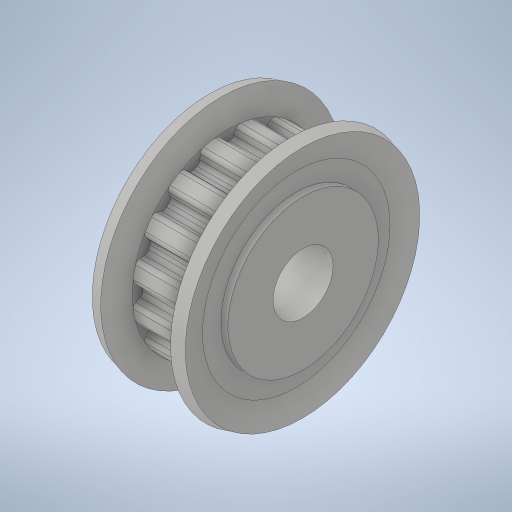
# Autodesk Inventor part: 3d_ATP16XL025-A-H8_b
Saved by Autodesk Inventor 2023 (Build 270158000, 158)
## iProperties
Category: PARTsolutions
Company: MISUMI
Created: 2023-01-14
Part Number: 3d_ATP16XL025-A-H8_b
Material: Generic
Catalog Web Link: www.cadenas.de
Description: ATP__XL025, ATP__XL031, ATP__ XL037, ATP__XL050, BTP__XL025, BTP__XL031, BTP__XL037, BTP__XL050, KTP__XL025, KTP__XL031, KTP__ XL037, KTP__XL050, NTP__XL025, NTP__XL031, NTP__ XL037, NTP__XL050, MTP__XL025, MTP__ XL037, MTP__XL050, MTPB__XL025, MTPB__ XL037, MTPB__XL050, MTPP__XL025, MTPP__ XL037, MTPP__XL050, STP__XL025, STP__ XL037, STP__XL050, KATP__XL025, KATP__XL031, KATP__ XL037, KATP__XL050, KKTP__XL025, KKTP__XL031, KKTP__ XL037, KKTP__XL050_body-Timing Pulleys XL Type
Vendor: MISUMI
Document SubType Name: Modeling
Designer: psAdmin
Manufacturer: MISUMI
Mass: 5.94338 g
Surface Area: 36.4815 cm^2
Volume: 5.94338 cm^3
Density: 1 g/cm^3
Appearance: PSOLRGB-175-175-175
PSOL_IDENT_0: {$CADENAS_DATA/23d-libs/misumi/metric/51_timing_pulleys/mtp_xl/mtp_xl.prj},873 {VTYP=3D},{NB=ATP16XL
PSOL_IDENT_1: 025-A-H8_b},{LINA=ATP16XL025-A-H8},{NN=ATP__XL025, ATP__XL031, ATP__ XL037, ATP__XL050, BTP__XL025,
PSOL_IDENT_2: BTP__XL031, BTP__XL037, BTP__XL050, KTP__XL025, KTP__XL031, KTP__ XL037, KTP__XL050, NTP__XL025, NTP
PSOL_IDENT_3: __XL031, NTP__ XL037, NTP__XL050, MTP__XL025, MTP__ XL037, MTP__XL050, MTPB__XL025, MTPB__ XL037, MT
PSOL_IDENT_4: PB__XL050, MTPP__XL025, MTPP__ XL037, MTPP__XL050, STP__XL025, STP__ XL037, STP__XL050, KATP__XL025,
PSOL_IDENT_5: KATP__XL031, KATP__ XL037, KATP__XL050, KKTP__XL025, KKTP__XL031, KKTP__ XL037, KKTP__XL050_body},{
PSOL_IDENT_6: DATE=25.04.2022 01:23:04},{GEOMDATE=17.11.2021 02:38:37},{VERSION=},{LINEID=30},{WBVAR=MATP,ST,TNW,P
PSOL_IDENT_7: S,SBS,DD,Z,J,Q,R,S,T,ALT1,ALT2,M,QSC,QFC,QTC,ALT3,K,KSC,KFC,KTC,ALT4,ZM,ZSC,ZFC,ZTC,ALT5,ALT6,ALT7,F
PSOL_IDENT_8: C,ALT8,SRG,ALT9,BTC,TL,ALT10,TPC,ALT11,BC,ALT12,SLH,ALT13,BN},{WBNUMERIC=DD,Z,J,Q,R,S,T,QSC,QFC,QTC,
PSOL_IDENT_9: K,KSC,KFC,KTC,ZSC,ZFC,ZTC,FC,SRG,BTC,TL,BC,SLH,BN}  {NB=ATP16XL025-A-H8_b},{LINA=ATP16XL025-A-H8},{K
PSOL_IDENT_10: T=DUMMY},{PN=ATP16XL025-A-H8},{TYPE=ATP},{MATP=A2017},{MATPALG= 'A2017','Aluminum Alloy 2000 series'
PSOL_IDENT_11: ,'S45C','1045 Carbon Steel Equivalent','SUS304','SUS304', 'A6000', '6000 Series Aluminum Alloy' },{S
PSOL_IDENT_12: T=CA},{STALG= 'CA','Clear Anodize','BA','Black Anodize','HAT','Hard Clear Anodize','ENP','Electroles
PSOL_IDENT_13: s Nickel Plating' },{NT=16},{TNW=XL025},{TNWALG= 'XL025','XL031','XL037','XL050' },{BW=6.4mm (1/4inc
PSOL_IDENT_14: h)},{PS=A},{PSALG= 'A','B' },{SBS=H},{SBSALG= 'H','Round Hole','P','Round Hole + Tap','N','New JIS K
PSOL_IDENT_15: eywayed Bore + Tap (Standard)','NK','New JIS Keywayed Bore + Tap (width 4.0mm, height 1.8mm)','C','O
PSOL_IDENT_16: ld JIS Keywayed Bore + Tap','V','Stepped Hole','Y','Both Ends Stepped Hole','WB','Double Stepped Hol
PSOL_IDENT_17: e' },{DD=8.00},{DDALG=[5:6/1],6.35,[7:12/1],12.7,[13:16/1]},{DDHA=[5:6/1],6.35,[7:12/1],12.7,[13:16/
PSOL_IDENT_18: 1]},{DDPA=[5:6/1],6.35,[7:12/1],12.7,[13:13/1]},{DDNA=[8:8/1],[10:13/1]},{DDNK=[10:10/1]},{DDCA=[10,
PSOL_IDENT_19: 12]},{DDVA=[5:6/1],6.35,[7:12/1],12.7,[13:14/1]},{DDY=[5:14/1]},{DDWB=[5:12/1]},{DDHB=},{DDPB=},{DDN
PSOL_IDENT_20: B=},{DDCB=},{DDVFB=},{Z=0},{ZALG=[0]},{ZMIN=10.000},{ZAMAX=16.000},{ZBMAX=0.000},{DDZ=8.000},{J=0.0}
PSOL_IDENT_21: ,{JALG=[0]},{JMIN=2.000},{JMAX=10.5},{JPN=},{Q=0},{QALG=[0]},{QRMIN=10.000},{QRMAX=16},{WBQMIN=12.00
PSOL_IDENT_22: 0},{R=0},{RALG=[0]},{WBRMAX=-2.000},{S=0.0},{SALG=[0]},{SMAX=6.5},{T=0.0},{TALG=[0]},{TMAX=8},{SBSPN=
PSOL_IDENT_23: -H8},{A=7.5},{W=12.5},{L=0},{PD=25.87},{OD=25.36},{D=0},{DALG=17.000},{DE=20},{F=32},{E=20},{TT=1.6}
PSOL_IDENT_24: ,{BBK=0.000},{TTK=0.0},{ALT1=},{ANG=112.500},{ALT1ALG= '','Not applicable' },{ALT1PN=},{ALT2=},{ALT2
PSOL_IDENT_25: ALG= '','Not applicable' },{M=N/A},{MALG= 'N/A' },{MFTALG= 'N/A' },{MSALG= 'N/A' },{M3D=0.000},{KDML=
PSOL_IDENT_26: 0.000},{ML=0.000},{MUL=0.000},{PITCH=0.000},{QSC=0.0},{QSCALG=0},{QFC=0.0},{QFCALG=0},{QTC=0.0},{QTC
PSOL_IDENT_27: ALG=0},{QPCDMIN=0.000},{QPCDMINALG=0.000},{QPCDMAX=16.000},{ALT2PN=},{TAP=0.000},{ALT3=},{ALT3ALG= ''
PSOL_IDENT_28: ,'Not applicable' },{K=0.0},{KALG=0},{KMIN=4.000},{KFTMAX=0.000},{KSMAX=0.000},{KSC=0.0},{KSCALG=0},
PSOL_IDENT_29: {KFC=0.0},{KFCALG=0},{KTC=0.0},{KTCALG=0},{KSCMIN=12.000},{KPCDMIN=12.000},{KPCDMAX=16.000},{ALT3PN=
PSOL_IDENT_30: },{ALT4=},{ALT4ALG= '','Not applicable' },{ALT4MIN=18.500},{ALT4MAX=9.500},{ZM=N/A},{ZMALG= 'N/A' },
PSOL_IDENT_31: {ZMFTALG= 'N/A' },{ZMSALG= 'N/A' },{ZMDD1=0.0},{ZMDD2=0.0},{ZMHH=0.0},{ZSC=0.0},{ZSCALG=[0]},{ZFC=0.
PSOL_IDENT_32: 0},{ZFCALG=[0]},{ZTC=0.0},{ZTCALG=[0]},{ZPCDMIN=0.000},{ZPCDMINALG=0.000},{ZPCDMAX=16.000},{ALT4PN=}
PSOL_IDENT_33: ,{ALT5=},{ALT5ALG= '','w/o Flange not Attached','NFC','with NFC (Flange not Attached)' },{ALT5PN=},{
PSOL_IDENT_34: ALT6=},{ALT6ALG= '','w/o Flange Attached on One Side Only','RFC','with RFC (Flange Attached on The B
PSOL_IDENT_35: oss Side Only)','LFC','with LFC (Flange Attached on The Opposite Side Only)' },{ALT6PN=},{ALT7=},{AL
PSOL_IDENT_36: T7ALG= '','w/o FC (Flange Cut)','FC','with FC (Flange Cut)' },{FC=0.0},{FCALG=0},{FCMIN=26.5},{FCMAX=
PSOL_IDENT_37: 30.0},{ALT7PN=},{ALT8=},{ALT8ALG= '','Not applicable' },{ALT8ALGALG=16.000},{ALT8DD2=0.000},{ALT8MM=
PSOL_IDENT_38: 0.000},{ALT8NN=0.000},{QC=0.000},{KC=0.000},{ZC=0.000},{SRG=0.0},{SRGALG=[0]},{SRGMAX=0.000},{DD2=0.
PSOL_IDENT_39: 0},{MM=0.00},{NN=0.00},{ALT8PN=},{ALT9=},{ALT9ALG= '','w/o BTC (Taper for Bearing Holder)','BTC','wi
PSOL_IDENT_40: th BTC (Taper for Bearing Holder)' },{BTC9=9.000},{TL9=1.000},{BTC=0},{BTCALG=[0]},{TL=0.0},{TLALG=0
PSOL_IDENT_41: },{TLMIN=1.000},{TLMAX=-13.000},{BTCL=0},{BTCD=0},{ALT9PN=},{WLBCTL=12.500},{ALT10=},{ALT10ALG= '','
PSOL_IDENT_42: Not applicable' },{TPC=N/A},{TPCALG= 'N/A' },{TPCM=4.000},{ALT10PN=},{ALT11=},{ALT11ALG= '','Not app
PSOL_IDENT_43: licable' },{BC=0.0},{BCALG=0},{BCMIN=3},{BCMAX=-13},{M1WBC=6.25},{ALT11PN=},{KTT=8.68},{ALT12=},{ALT
PSOL_IDENT_44: 12ALG= '','Not applicable' },{SLHALG=[0]},{SLH=0},{ALT12PN=},{ALT13=},{ALT13ALG= '', 'Not applicable'
PSOL_IDENT_45: },{BN=0.0},{BNALG=0},{BNMIN=-12},{BNMAX=-2.5},{ALT13PN=},{AC=-},{M1=4.000},{M1L=3.000},{KEYA=0.000}
PSOL_IDENT_46: ,{KEYB=0.000},{KEYM=0.000}
NB: ATP16XL025-A-H8_b
NN: 0
NT: 16
NBSYN: $PN._b
LINA: ATP16XL025-A-H8
CATALOG: Misumi
PN: ATP16XL025-A-H8
MATP: Aluminum Alloy 2000 series
ST: Clear Anodize
TNW: XL025
BW: 6.4mm (1/4inch)
PS: A
SBS: Round Hole
DD: 8
Z: 0
J: 0
Q: 0
R: 0
S: 0
T: 0
A: 7.5
W: 12.5
L: 0
PD: 25.87
OD: 25.36
D: 0
F: 32
E: 20
TT: 1.6
ALT1: Not applicable
ALT2: Not applicable
M: N/A
QSC: 0
QFC: 0
QTC: 0
ALT3: Not applicable
K: 0
KSC: 0
KFC: 0
KTC: 0
ALT4: Not applicable
ZM: N/A
ZMDD1: 0
ZMDD2: 0
ZMHH: 0
ZSC: 0
ZFC: 0
ZTC: 0
ALT5: w/o Flange not Attached
ALT6: w/o Flange Attached on One Side Only
ALT7: w/o FC (Flange Cut)
FC: 0
ALT8: Not applicable
SRG: 0
DD2: 0
MM: 0
ALT9: w/o BTC (Taper for Bearing Holder)
BTC: 0
TL: 0
BTCL: 0
BTCD: 0
ALT10: Not applicable
TPC: N/A
ALT11: Not applicable
BC: 0
ALT12: Not applicable
SLH: 0
ALT13: Not applicable
BN: 0
AC: -
SUPPLIER: MISUMI
ARTICLENO: ATP16XL025-A-H8_b
BOMINFO: ATP16XL025-A-H8
CREATOR: CADENAS GmbH
Title: ATP16XL025-A-H8
Author: Cadenas PARTsolutions
Comments: Timing Pulleys XL Type
Autodesk Inventor part; units mm, degrees
ref_plane "YZ Plane" through (0, 0, 0) normal (1, 0, 0) x (0, 1, 0)
ref_plane "XZ Plane" through (0, 0, 0) normal (0, 1, 0) x (-1, 0, 0)
ref_plane "XY Plane" through (0, 0, 0) normal (0, 0, 1) x (1, 0, 0)
sketch "_____2" plane through (0, 0, 0) normal (0, 0, 1) x (1, 0, 0)
  line L0 (12.5, 0) -> (0, 0)
  line L1 (0, 0) -> (0, 10)
  line L2 (0, 10) -> (0.9, 10)
  line L3 (0.9, 10) -> (0.9, 12.469356)
  line L4 (0.9, 12.469356) -> (0.064927, 15.58589)
  line L5 (0.064927, 15.58589) -> (1.610409, 16)
  line L6 (1.610409, 16) -> (2.5, 12.68)
  line L7 (2.5, 12.68) -> (10, 12.68)
  line L8 (10, 12.68) -> (10.889591, 16)
  line L9 (10.889591, 16) -> (12.435073, 15.58589)
  line L10 (12.435073, 15.58589) -> (11.6, 12.469356)
  line L11 (11.6, 12.469356) -> (11.6, 10)
  line L12 (11.6, 10) -> (12.5, 10)
  line L13 (12.5, 10) -> (12.5, 0)
  line L14 (12.5, 0) -> (0, 0)
  constraints: 30 end point
revolve "Revolution1" add sketch "_____2" angle 360 about axis through (12.5, 0, 0) along (1, 0, 0)
sketch "Sketch2" plane through (12.5, 0, 0) normal (1, 0, 0) x (0, 0, -1)
  point P0 (0, 0)
hole "Hole1" at (12.5, 0, 0) direction (-1, 0, 0) diameter 8 depth 12.5
sketch "_____6" plane through (2.5, 0, 0) normal (1, 0, 0) x (0, 0, -1)
  arc A0 (-12.686458, 2.523493) -> (-12.686458, -2.523493) centre (0, 0) ccw
  arc A1 (-12.686458, -2.523493) -> (-10.755059, -7.186301) centre (0, 0) ccw
  arc A2 (-10.755059, -7.186301) -> (-7.186301, -10.755059) centre (0, 0) ccw
  arc A3 (-7.186301, -10.755059) -> (-2.523493, -12.686458) centre (0, 0) ccw
  arc A4 (-2.523493, -12.686458) -> (2.523493, -12.686458) centre (0, 0) ccw
  arc A5 (2.523493, -12.686458) -> (7.186301, -10.755059) centre (0, 0) ccw
  arc A6 (7.186301, -10.755059) -> (10.755059, -7.186301) centre (0, 0) ccw
  arc A7 (10.755059, -7.186301) -> (12.686458, -2.523493) centre (0, 0) ccw
  arc A8 (12.686458, -2.523493) -> (12.686458, 2.523493) centre (0, 0) ccw
  arc A9 (12.686458, 2.523493) -> (10.755059, 7.186301) centre (0, 0) ccw
  arc A10 (10.755059, 7.186301) -> (7.186301, 10.755059) centre (0, 0) ccw
  arc A11 (7.186301, 10.755059) -> (2.523493, 12.686458) centre (0, 0) ccw
  arc A12 (2.523493, 12.686458) -> (-2.523493, 12.686458) centre (0, 0) ccw
  arc A13 (-2.523493, 12.686458) -> (-7.186301, 10.755059) centre (0, 0) ccw
  arc A14 (-7.186301, 10.755059) -> (-10.755059, 7.186301) centre (0, 0) ccw
  arc A15 (-10.755059, 7.186301) -> (-12.686458, 2.523493) centre (0, 0) ccw
  arc A16 (-12.216815, -1.080185) -> (-12.563409, -1.715564) centre (-11.959018, -1.633033) ccw
  arc A17 (-12.563409, -1.715564) -> (-12.436357, -2.473745) centre (0, 0) ccw
  arc A18 (-12.436357, -2.473745) -> (-12.263594, -3.222834) centre (0, 0) ccw
  arc A19 (-12.263594, -3.222834) -> (-11.700234, -3.677212) centre (-11.673626, -3.067792) ccw
  line L0 (-11.700234, -3.677212) -> (-11.052822, -3.705478)
  arc A20 (-10.511015, -4.093528) -> (-11.052822, -3.705478) centre (-11.079429, -4.314898) ccw
  arc A21 (-10.511015, -4.093528) -> (-10.326971, -4.537849) centre (0, 0) ccw
  arc A22 (-10.435694, -5.195356) -> (-10.326971, -4.537849) centre (-10.885433, -4.783246) ccw
  line L1 (-10.435694, -5.195356) -> (-10.873496, -5.673133)
  arc A23 (-10.873496, -5.673133) -> (-10.950558, -6.392783) centre (-10.423757, -6.085244) ccw
  arc A24 (-10.950558, -6.392783) -> (-10.543035, -7.044631) centre (0, 0) ccw
  arc A25 (-10.543035, -7.044631) -> (-10.096758, -7.670585) centre (0, 0) ccw
  arc A26 (-10.096758, -7.670585) -> (-9.402399, -7.874786) centre (-9.611031, -7.301574) ccw
  line L2 (-9.402399, -7.874786) -> (-8.79345, -7.653147)
  arc A27 (-8.144386, -7.804318) -> (-8.79345, -7.653147) centre (-8.584818, -8.22636) ccw
  arc A28 (-8.144386, -7.804318) -> (-7.804318, -8.144386) centre (0, 0) ccw
  arc A29 (-7.653147, -8.79345) -> (-7.804318, -8.144386) centre (-8.22636, -8.584818) ccw
  line L3 (-7.653147, -8.79345) -> (-7.874786, -9.402399)
  arc A30 (-7.874786, -9.402399) -> (-7.670585, -10.096758) centre (-7.301574, -9.611031) ccw
  arc A31 (-7.670585, -10.096758) -> (-7.044631, -10.543035) centre (0, 0) ccw
  arc A32 (-7.044631, -10.543035) -> (-6.392783, -10.950558) centre (0, 0) ccw
  arc A33 (-6.392783, -10.950558) -> (-5.673133, -10.873496) centre (-6.085244, -10.423757) ccw
  line L4 (-5.673133, -10.873496) -> (-5.195356, -10.435694)
  arc A34 (-4.537848, -10.326971) -> (-5.195356, -10.435694) centre (-4.783246, -10.885433) ccw
  arc A35 (-4.537848, -10.326971) -> (-4.093528, -10.511015) centre (0, 0) ccw
  arc A36 (-3.705478, -11.052822) -> (-4.093528, -10.511015) centre (-4.314898, -11.079429) ccw
  line L5 (-3.705478, -11.052822) -> (-3.677212, -11.700234)
  arc A37 (-3.677212, -11.700234) -> (-3.222834, -12.263594) centre (-3.067792, -11.673626) ccw
  arc A38 (-3.222834, -12.263594) -> (-2.473745, -12.436357) centre (0, 0) ccw
  arc A39 (-2.473745, -12.436357) -> (-1.715564, -12.563409) centre (0, 0) ccw
  arc A40 (-1.715564, -12.563409) -> (-1.080185, -12.216815) centre (-1.633033, -11.959018) ccw
  line L6 (-1.080185, -12.216815) -> (-0.806316, -11.629501)
  arc A41 (-0.240464, -11.277437) -> (-0.806316, -11.629501) centre (-0.253468, -11.887298) ccw
  arc A42 (-0.240464, -11.277437) -> (0.240464, -11.277437) centre (0, 0) ccw
  arc A43 (0.806316, -11.629501) -> (0.240464, -11.277437) centre (0.253468, -11.887298) ccw
  line L7 (0.806316, -11.629501) -> (1.080185, -12.216815)
  arc A44 (1.080185, -12.216815) -> (1.715564, -12.563409) centre (1.633033, -11.959018) ccw
  arc A45 (1.715564, -12.563409) -> (2.473745, -12.436357) centre (0, 0) ccw
  arc A46 (2.473745, -12.436357) -> (3.222834, -12.263594) centre (0, 0) ccw
  arc A47 (3.222834, -12.263594) -> (3.677212, -11.700234) centre (3.067792, -11.673626) ccw
  line L8 (3.677212, -11.700234) -> (3.705478, -11.052822)
  arc A48 (4.093528, -10.511015) -> (3.705478, -11.052822) centre (4.314898, -11.079429) ccw
  arc A49 (4.093528, -10.511015) -> (4.537849, -10.326971) centre (0, 0) ccw
  arc A50 (5.195356, -10.435694) -> (4.537849, -10.326971) centre (4.783246, -10.885433) ccw
  line L9 (5.195356, -10.435694) -> (5.673133, -10.873496)
  arc A51 (5.673133, -10.873496) -> (6.392783, -10.950558) centre (6.085244, -10.423757) ccw
  arc A52 (6.392783, -10.950558) -> (7.044631, -10.543035) centre (0, 0) ccw
  arc A53 (7.044631, -10.543035) -> (7.670585, -10.096758) centre (0, 0) ccw
  arc A54 (7.670585, -10.096758) -> (7.874786, -9.402399) centre (7.301574, -9.611031) ccw
  line L10 (7.874786, -9.402399) -> (7.653147, -8.79345)
  arc A55 (7.804318, -8.144386) -> (7.653147, -8.79345) centre (8.22636, -8.584818) ccw
  arc A56 (7.804318, -8.144386) -> (8.144386, -7.804318) centre (0, 0) ccw
  arc A57 (8.79345, -7.653147) -> (8.144386, -7.804318) centre (8.584818, -8.22636) ccw
  line L11 (8.79345, -7.653147) -> (9.402399, -7.874786)
  arc A58 (9.402399, -7.874786) -> (10.096758, -7.670585) centre (9.611031, -7.301574) ccw
  arc A59 (10.096758, -7.670585) -> (10.543035, -7.044631) centre (0, 0) ccw
  arc A60 (10.543035, -7.044631) -> (10.950558, -6.392783) centre (0, 0) ccw
  arc A61 (10.950558, -6.392783) -> (10.873496, -5.673133) centre (10.423757, -6.085244) ccw
  line L12 (10.873496, -5.673133) -> (10.435694, -5.195356)
  arc A62 (10.326971, -4.537848) -> (10.435694, -5.195356) centre (10.885433, -4.783246) ccw
  arc A63 (10.326971, -4.537848) -> (10.511015, -4.093528) centre (0, 0) ccw
  arc A64 (11.052822, -3.705478) -> (10.511015, -4.093528) centre (11.079429, -4.314898) ccw
  line L13 (11.052822, -3.705478) -> (11.700234, -3.677212)
  arc A65 (11.700234, -3.677212) -> (12.263594, -3.222834) centre (11.673626, -3.067792) ccw
  arc A66 (12.263594, -3.222834) -> (12.436357, -2.473745) centre (0, 0) ccw
  arc A67 (12.436357, -2.473745) -> (12.563409, -1.715564) centre (0, 0) ccw
  arc A68 (12.563409, -1.715564) -> (12.216815, -1.080185) centre (11.959018, -1.633033) ccw
  line L14 (12.216815, -1.080185) -> (11.629501, -0.806316)
  arc A69 (11.277437, -0.240464) -> (11.629501, -0.806316) centre (11.887298, -0.253468) ccw
  arc A70 (11.277437, -0.240464) -> (11.277437, 0.240464) centre (0, 0) ccw
  arc A71 (11.629501, 0.806316) -> (11.277437, 0.240464) centre (11.887298, 0.253468) ccw
  line L15 (11.629501, 0.806316) -> (12.216815, 1.080185)
  arc A72 (12.216815, 1.080185) -> (12.563409, 1.715564) centre (11.959018, 1.633033) ccw
  arc A73 (12.563409, 1.715564) -> (12.436357, 2.473745) centre (0, 0) ccw
  arc A74 (12.436357, 2.473745) -> (12.263594, 3.222834) centre (0, 0) ccw
  arc A75 (12.263594, 3.222834) -> (11.700234, 3.677212) centre (11.673626, 3.067792) ccw
  line L16 (11.700234, 3.677212) -> (11.052822, 3.705478)
  arc A76 (10.511015, 4.093528) -> (11.052822, 3.705478) centre (11.079429, 4.314898) ccw
  arc A77 (10.511015, 4.093528) -> (10.326971, 4.537848) centre (0, 0) ccw
  arc A78 (10.435694, 5.195356) -> (10.326971, 4.537848) centre (10.885433, 4.783246) ccw
  line L17 (10.435694, 5.195356) -> (10.873496, 5.673133)
  arc A79 (10.873496, 5.673133) -> (10.950558, 6.392783) centre (10.423757, 6.085244) ccw
  arc A80 (10.950558, 6.392783) -> (10.543035, 7.044631) centre (0, 0) ccw
  arc A81 (10.543035, 7.044631) -> (10.096758, 7.670585) centre (0, 0) ccw
  arc A82 (10.096758, 7.670585) -> (9.402399, 7.874786) centre (9.611031, 7.301574) ccw
  line L18 (9.402399, 7.874786) -> (8.79345, 7.653147)
  arc A83 (8.144386, 7.804318) -> (8.79345, 7.653147) centre (8.584818, 8.22636) ccw
  arc A84 (8.144386, 7.804318) -> (7.804318, 8.144386) centre (0, 0) ccw
  arc A85 (7.653147, 8.79345) -> (7.804318, 8.144386) centre (8.22636, 8.584818) ccw
  line L19 (7.653147, 8.79345) -> (7.874786, 9.402399)
  arc A86 (7.874786, 9.402399) -> (7.670585, 10.096758) centre (7.301574, 9.611031) ccw
  arc A87 (7.670585, 10.096758) -> (7.044631, 10.543035) centre (0, 0) ccw
  arc A88 (7.044631, 10.543035) -> (6.392783, 10.950558) centre (0, 0) ccw
  arc A89 (6.392783, 10.950558) -> (5.673133, 10.873496) centre (6.085244, 10.423757) ccw
  line L20 (5.673133, 10.873496) -> (5.195356, 10.435694)
  arc A90 (4.537848, 10.326971) -> (5.195356, 10.435694) centre (4.783246, 10.885433) ccw
  arc A91 (4.537848, 10.326971) -> (4.093528, 10.511015) centre (0, 0) ccw
  arc A92 (3.705478, 11.052822) -> (4.093528, 10.511015) centre (4.314898, 11.079429) ccw
  line L21 (3.705478, 11.052822) -> (3.677212, 11.700234)
  arc A93 (3.677212, 11.700234) -> (3.222834, 12.263594) centre (3.067792, 11.673626) ccw
  arc A94 (3.222834, 12.263594) -> (2.473745, 12.436357) centre (0, 0) ccw
  arc A95 (2.473745, 12.436357) -> (1.715564, 12.563409) centre (0, 0) ccw
  arc A96 (1.715564, 12.563409) -> (1.080185, 12.216815) centre (1.633033, 11.959018) ccw
  line L22 (1.080185, 12.216815) -> (0.806316, 11.629501)
  arc A97 (0.240465, 11.277437) -> (0.806316, 11.629501) centre (0.253468, 11.887298) ccw
  arc A98 (0.240465, 11.277437) -> (-0.240465, 11.277437) centre (0, 0) ccw
  arc A99 (-0.806316, 11.629501) -> (-0.240465, 11.277437) centre (-0.253468, 11.887298) ccw
  line L23 (-0.806316, 11.629501) -> (-1.080185, 12.216815)
  arc A100 (-1.080185, 12.216815) -> (-1.715564, 12.563409) centre (-1.633033, 11.959018) ccw
  arc A101 (-1.715564, 12.563409) -> (-2.473745, 12.436357) centre (0, 0) ccw
  arc A102 (-2.473745, 12.436357) -> (-3.222834, 12.263594) centre (0, 0) ccw
  arc A103 (-3.222834, 12.263594) -> (-3.677212, 11.700234) centre (-3.067792, 11.673626) ccw
  line L24 (-3.677212, 11.700234) -> (-3.705478, 11.052822)
  arc A104 (-4.093528, 10.511015) -> (-3.705478, 11.052822) centre (-4.314898, 11.079429) ccw
  arc A105 (-4.093528, 10.511015) -> (-4.537849, 10.326971) centre (0, 0) ccw
  arc A106 (-5.195356, 10.435694) -> (-4.537849, 10.326971) centre (-4.783246, 10.885433) ccw
  line L25 (-5.195356, 10.435694) -> (-5.673133, 10.873496)
  arc A107 (-5.673133, 10.873496) -> (-6.392783, 10.950558) centre (-6.085244, 10.423757) ccw
  arc A108 (-6.392783, 10.950558) -> (-7.044631, 10.543035) centre (0, 0) ccw
  arc A109 (-7.044631, 10.543035) -> (-7.670585, 10.096758) centre (0, 0) ccw
  arc A110 (-7.670585, 10.096758) -> (-7.874786, 9.402399) centre (-7.301574, 9.611031) ccw
  line L26 (-7.874786, 9.402399) -> (-7.653147, 8.79345)
  arc A111 (-7.804318, 8.144386) -> (-7.653147, 8.79345) centre (-8.22636, 8.584818) ccw
  arc A112 (-7.804318, 8.144386) -> (-8.144386, 7.804318) centre (0, 0) ccw
  arc A113 (-8.79345, 7.653147) -> (-8.144386, 7.804318) centre (-8.584818, 8.22636) ccw
  line L27 (-8.79345, 7.653147) -> (-9.402399, 7.874786)
  arc A114 (-9.402399, 7.874786) -> (-10.096758, 7.670585) centre (-9.611031, 7.301574) ccw
  arc A115 (-10.096758, 7.670585) -> (-10.543035, 7.044631) centre (0, 0) ccw
  arc A116 (-10.543035, 7.044631) -> (-10.950558, 6.392783) centre (0, 0) ccw
  arc A117 (-10.950558, 6.392783) -> (-10.873496, 5.673133) centre (-10.423757, 6.085244) ccw
  line L28 (-10.873496, 5.673133) -> (-10.435694, 5.195356)
  arc A118 (-10.326971, 4.537848) -> (-10.435694, 5.195356) centre (-10.885433, 4.783246) ccw
  arc A119 (-10.326971, 4.537848) -> (-10.511015, 4.093528) centre (0, 0) ccw
  arc A120 (-11.052822, 3.705478) -> (-10.511015, 4.093528) centre (-11.079429, 4.314898) ccw
  line L29 (-11.052822, 3.705478) -> (-11.700234, 3.677212)
  arc A121 (-11.700234, 3.677212) -> (-12.263594, 3.222834) centre (-11.673626, 3.067792) ccw
  arc A122 (-12.263594, 3.222834) -> (-12.436357, 2.473745) centre (0, 0) ccw
  arc A123 (-12.436357, 2.473745) -> (-12.563409, 1.715564) centre (0, 0) ccw
  arc A124 (-12.563409, 1.715564) -> (-12.216815, 1.080185) centre (-11.959018, 1.633033) ccw
  line L30 (-12.216815, 1.080185) -> (-11.629501, 0.806316)
  arc A125 (-11.277437, 0.240465) -> (-11.629501, 0.806316) centre (-11.887298, 0.253468) ccw
  arc A126 (-11.277437, 0.240465) -> (-11.277437, -0.240465) centre (0, 0) ccw
  arc A127 (-11.629501, -0.806316) -> (-11.277437, -0.240465) centre (-11.887298, -0.253468) ccw
  line L31 (-11.629501, -0.806316) -> (-12.216815, -1.080185)
  constraints: 256 point on circle, 128 centre point, 64 end point
extrude "Extrusion1" cut sketch "_____6" along normal blind 7.5
body "Solid1"
